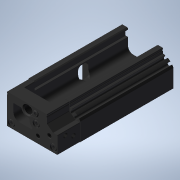
# Autodesk Inventor part: DGSL-12---(50-0-0-30-zr)
Saved by Autodesk Inventor 2021 (Build 250183000, 183)
## iProperties
Created: 2026-04-25
Part Number: DGSL-12---(50-0-0-30-zr)
Material: Generic
Catalog Web Link: www.3dfindit.com
Description: DGSL-(ZR)-Mini slide, cylinder
Vendor: FESTO
Document SubType Name: Modeling
Designer: psAdmin
Manufacturer: FESTO
Mass: 154.278 g
Surface Area: 450.594 cm^2
Volume: 154.278 cm^3
Density: 1 g/cm^3
Appearance: PSOLRGB-176-176-176
Category: PARTsolutions
Company: FESTO
Title: DGSL-12-50-0-0-3
Author: Cadenas PARTsolutions
Comments: Mini slide, cylinder
PSOL_IDENT_0: {$CADENAS_DATA/23d-libs/festo/parts/d/dgsl/parts/dgsl_zylinder.prj},221 {VTYP=3D},{NB=DGSL-12---(50-
PSOL_IDENT_1: 0-0-30-zr)},{LINA=DGSL-12-50-0-0-3},{NN=DGSL-(ZR)},{DATE=08.01.2026 09:23:11},{GEOMDATE=08.01.2026 0
PSOL_IDENT_2: 9:23:00},{VERSION=},{LINEID=110},{WBVAR=TYP2,HUB,FE,EL,DA,HGO},{WBNUMERIC=HUB,FE,EL,DA,HGO}  {NB=DGS
PSOL_IDENT_3: L-12---(50-0-0-30-zr)},{LINA=DGSL-12-50-0-0-3},{KT=DUMMY},{TYP=DGSL-12},{TYP2=},{TYP22=},{KDM=16},{E
PSOL_IDENT_4: E=M5},{KDM2=12},{PS=A},{ZB=24.000},{B4=34.000},{HUB=50},{FE=0},{EL=0},{DA=3},{OFFX=-0.500},{OFFY=-1.
PSOL_IDENT_5: 500},{LAOFF=0.500},{T1=8.700},{T11=14.000},{T1H=10.800},{T1R=4.000},{LA=10.000},{LA2=4.500},{LAN=5.0
PSOL_IDENT_6: 00},{LAH=1.600},{LAH2=5.600},{LAH3=11.300},{LAD1=7.000},{LAD2=9.000},{LAD3=5.500},{L=108.6},{LD=26.0
PSOL_IDENT_7: 00},{LD1=11.900},{B=59.000},{B0=45.100},{B1=23.800},{B1A=24.970},{B1B=9.250},{B2=36.700},{B3=50.000}
PSOL_IDENT_8: ,{B6=5.000},{H0=14.300},{H1=27.700},{H1A=27.800},{H1B=5.000},{H2=8.000},{H3=15.100},{H4=18.800},{H5=
PSOL_IDENT_9: 24.900},{H6=5.000},{H16=5.000},{L2=26.85},{L2P=26.900},{L2P1=25.700},{L2Y3=26.850},{L5=82.4},{L6=0},
PSOL_IDENT_10: {L7=0},{L8=12.000},{D1N=10},{D1B=9.100},{D2N=5.000},{D3N=5.000},{D4N=4.300},{D4N2=8.000},{D4HEX=3.00
PSOL_IDENT_11: 0},{D4HEXR=1.800},{D6A=8.000},{D6B=4.300},{KSD1=16.500},{KSD=6.000},{SH1=10.250},{SH2=15.250},{SL1=1
PSOL_IDENT_12: 8.5},{ST1=24.000},{ST11=5.500},{SDN1=5.000},{SL2=9.000},{ST2=12.800},{ST22=5.500},{SDN2=5.000},{E3H=
PSOL_IDENT_13: 14.800},{E3B=0},{E3B1=10.500},{E3B2=19.900},{E3L=10.300},{E3D=16.000},{E3X=0.500},{SDDNP=10.000},{SD
PSOL_IDENT_14: DNY3=10.000},{D1K=8.917},{D1P=1.000},{KPX=3.600},{KPL=18.000},{KPR=3.000},{KPH=24.000},{ANSOFF=0.500
PSOL_IDENT_15: },{SH=59.000},{KEH=10.600},{KEB=5.000},{KED=6.000},{KEN=6.000},{KENS=3.000},{KENT=2.000},{BND=3.000}
PSOL_IDENT_16: ,{BNT=6.000},{BNT2=8.000},{BNP=30.800},{BNP2=10.000},{FI=4.600},{FD=8.000},{FP1=54.000},{FP2=5.000},
PSOL_IDENT_17: {FP3=5.000},{DK=7.000},{K=4.000},{S=3.000},{T=2.000},{RD=4.600},{L100=1.200},{L101=9.500},{H101=14.6
PSOL_IDENT_18: 00},{L102=22.800},{H102=7.500},{L103=5.500},{L104=9.500},{L105=5.500},{L106=18.400},{L107=7.000},{L1
PSOL_IDENT_19: 08=9.400},{D107=4.000},{L109=6.000},{HUBSTOFF=1.600},{HUBCORR=1.600},{L110=5.000},{L111=3.000},{D111=
PSOL_IDENT_20: 8.080},{GEHL=60.000},{HGO=0},{SENX=49.203},{SENY=23.978},{SENX2=53.110},{SENY2=21.097},{SENW=153.500
PSOL_IDENT_21: },{SENW2=133.000}
NB: DGSL-12---(50-0-0-30-zr)
NN: DGSL-(ZR)
NT: Mini slide, cylinder
NBSYN: $TYP.$TYP22.---($HUB.-$FE.-$EL.-$DA.$HGO.-zr)
LINA: DGSL-12-50-0-0-3
CATALOG: Festo
TYP: DGSL-12
KDM: 16
EE: M5
ZB: 24
HUB: 50
FE: -
EL: -
DA: Y3
T11: 14
ST11: 5.5
ST22: 5.5
D1K: 8.917
D1P: 1
ANSOFF: 0.5
SH: 59
KEH: 10.6
KEB: 5
KED: 6
KEN: 6
KENS: 3
KENT: 2
BND: 3
BNT: 6
BNT2: 8
BNP: 30.8
BNP2: 10
FI: 4.6
FD: 8
FP1: 54
FP2: 5
FP3: 5
DK: 7
K: 4
S: 3
T: 2
RD: 4.6
L100: 1.2
L101: 9.5
H101: 14.6
L102: 22.8
H102: 7.5
L103: 5.5
L104: 9.5
L105: 5.5
L106: 18.4
L107: 7
L108: 9.4
D107: 4
L109: 6
HUBSTOFF: 1.6
L110: 5
L111: 3
D111: 8.08
GEHL: 60
HGO: 0
SENX: 49.203
SENY: 23.978
SENX2: 53.11
SENY2: 21.097
SENW: 153.5
SENW2: 133
SUPPLIER: FESTO
ARTICLENO: DGSL-12---(50-0-0-30-zr)
BOMINFO: DGSL-12-50-0-0-3
CREATOR: CADENAS GmbH
Autodesk Inventor part; units mm, degrees
sketch "Skizze_Deckelprofil_12" plane through (0, 0, 0) normal (0, 0, 1) x (1, 0, 0)
  arc A0 (0, 0.5) -> (0.5, 0) centre (0.5, 0.5) ccw
  line L0 (0.5, 0) -> (58.5, 0)
  arc A1 (58.5, 0) -> (59, 0.5) centre (58.5, 0.5) ccw
  line L1 (59, 0.5) -> (59, 19.35)
  arc A2 (59, 19.35) -> (58.5, 19.85) centre (58.5, 19.35) ccw
  line L2 (58.5, 19.85) -> (54.1325, 19.85)
  arc A3 (53.7137, 19.9891) -> (54.1325, 19.85) centre (54.1325, 20.55) ccw
  line L3 (53.7137, 19.9891) -> (46.8812, 25.0912)
  arc A4 (46.6, 25.6521) -> (46.8812, 25.0912) centre (47.3, 25.6521) ccw
  line L4 (46.6, 25.6521) -> (46.6, 31.5253)
  arc A5 (46.6, 31.5253) -> (46.5167, 31.6878) centre (46.4, 31.5253) ccw
  arc A6 (46.5167, 33.3122) -> (46.5167, 31.6878) centre (47.1, 32.5) ccw
  arc A7 (46.5167, 33.3122) -> (46.6, 33.4747) centre (46.4, 33.4747) ccw
  line L5 (46.6, 33.4747) -> (46.6, 34.2)
  arc A8 (46.6, 34.2) -> (46.1, 34.7) centre (46.1, 34.2) ccw
  line L6 (46.1, 34.7) -> (0.5, 34.7)
  arc A9 (0.5, 34.7) -> (0, 34.2) centre (0.5, 34.2) ccw
  line L7 (0, 34.2) -> (0, 33.4747)
  arc A10 (0, 33.4747) -> (0.0833, 33.3122) centre (0.2, 33.4747) ccw
  arc A11 (0.0833, 31.6878) -> (0.0833, 33.3122) centre (-0.5, 32.5) ccw
  arc A12 (0.0833, 31.6878) -> (0, 31.5253) centre (0.2, 31.5253) ccw
  line L8 (0, 31.5253) -> (0, 0.5)
  arc A13 (7.5, 17.8) -> (14.5, 10.8) centre (14.5, 17.8) ccw
  line L9 (14.5, 10.8) -> (28.9, 10.8)
  arc A14 (28.9, 10.8) -> (29.5, 11.4) centre (28.9, 11.4) ccw
  line L10 (29.5, 11.4) -> (29.5, 12.7814)
  arc A15 (29.5, 12.7814) -> (29.2417, 13.2746) centre (28.9, 12.7814) ccw
  arc A16 (26.4, 18.7) -> (29.2417, 13.2746) centre (33, 18.7) ccw
  line L11 (26.4, 18.7) -> (26.4, 19.8616)
  arc A17 (26.4, 19.8616) -> (25.2, 20.8414) centre (25.4, 19.8616) ccw
  arc A18 (16.9377, 26.3184) -> (25.2, 20.8414) centre (23.8, 27.7) ccw
  arc A19 (16.9377, 26.3184) -> (16.3495, 26.8) centre (16.3495, 26.2) ccw
  line L12 (16.3495, 26.8) -> (8.1, 26.8)
  arc A20 (8.1, 26.8) -> (7.5, 26.2) centre (8.1, 26.2) ccw
  line L13 (7.5, 26.2) -> (7.5, 17.8)
  constraints: 42 point on circle, 28 end point, 21 centre point
extrude "Extrusion1" add sketch "Skizze_Deckelprofil_12" along normal blind 26
sketch "Skizze_Gehaeuseprofil_12" plane through (0, 0, 0) normal (0, 0, 1) x (1, 0, 0)
  line L0 (-0.5, 0.3) -> (0, -0.2)
  line L1 (0, -0.2) -> (5.65, -0.2)
  line L2 (5.65, -0.2) -> (5.95, -0.5)
  line L3 (5.95, -0.5) -> (41.2, -0.5)
  line L4 (41.2, -0.5) -> (41.5, -0.2)
  line L5 (41.5, -0.2) -> (59, -0.2)
  line L6 (59, -0.2) -> (59.5, 0.3)
  line L7 (59.5, 0.3) -> (59.5, 20.9212)
  arc A0 (59.5, 20.9212) -> (59.4448, 21.1495) centre (59, 20.9212) ccw
  arc A1 (59.4448, 21.1495) -> (58.0866, 23.3179) centre (46.1, 14.3) ccw
  arc A2 (58.0866, 23.3179) -> (57.7956, 23.3486) centre (57.9268, 23.1976) ccw
  line L8 (57.7956, 23.3486) -> (56.2727, 22.0247)
  arc A3 (56.2727, 22.0247) -> (56.2529, 21.7426) centre (56.4039, 21.8738) ccw
  arc A4 (56.2155, 21.4467) -> (56.2529, 21.7426) centre (56.102, 21.6114) ccw
  line L9 (56.2155, 21.4467) -> (55.4047, 20.8876)
  arc A5 (53.0577, 23.5876) -> (55.4047, 20.8876) centre (54.3829, 22.3695) ccw
  line L10 (53.0577, 23.5876) -> (53.7241, 24.3127)
  arc A6 (54.0223, 24.3086) -> (53.7241, 24.3127) centre (53.8714, 24.1774) ccw
  arc A7 (54.0223, 24.3086) -> (54.3045, 24.2889) centre (54.1733, 24.4398) ccw
  line L11 (54.3045, 24.2889) -> (55.7128, 25.513)
  arc A8 (55.7128, 25.513) -> (55.7097, 25.8176) centre (55.5815, 25.664) ccw
  arc A9 (55.7097, 25.8176) -> (52.9206, 27.6596) centre (46.1, 14.3) ccw
  arc A10 (52.9206, 27.6596) -> (52.647, 27.5628) centre (52.8297, 27.4815) ccw
  line L12 (52.647, 27.5628) -> (51.9613, 26.0228)
  arc A11 (51.9613, 26.0228) -> (52.0626, 25.7587) centre (52.144, 25.9414) ccw
  arc A12 (52.1538, 25.4747) -> (52.0626, 25.7587) centre (51.9813, 25.576) ccw
  line L13 (52.1538, 25.4747) -> (51.6552, 24.6254)
  arc A13 (48.387, 26.0805) -> (51.6552, 24.6254) centre (50.1029, 25.5366) ccw
  line L14 (48.387, 26.0805) -> (48.6846, 27.0193)
  arc A14 (48.9566, 27.1416) -> (48.6846, 27.0193) centre (48.8752, 26.9589) ccw
  arc A15 (48.9566, 27.1416) -> (49.2206, 27.243) centre (49.0379, 27.3243) ccw
  line L15 (49.2206, 27.243) -> (49.8202, 28.5897)
  arc A16 (49.8202, 28.5897) -> (49.6853, 28.8652) centre (49.6375, 28.671) ccw
  arc A17 (49.6853, 28.8652) -> (47.3745, 29.2458) centre (46.1, 14.3) ccw
  arc A18 (47.1, 29.5447) -> (47.3745, 29.2458) centre (47.4, 29.5447) ccw
  line L16 (47.1, 29.5447) -> (47.1, 31.6225)
  arc A19 (47.1, 31.6225) -> (46.9444, 31.8175) centre (46.9, 31.6225) ccw
  arc A20 (46.9444, 33.1825) -> (46.9444, 31.8175) centre (47.1, 32.5) ccw
  arc A21 (46.9444, 33.1825) -> (47.1, 33.3775) centre (46.9, 33.3775) ccw
  line L17 (47.1, 33.3775) -> (47.1, 34.5)
  arc A22 (47.1, 34.5) -> (46.6, 35) centre (46.6, 34.5) ccw
  line L18 (46.6, 35) -> (41.7124, 35)
  line L19 (41.7124, 35) -> (40.5, 34.3)
  line L20 (40.5, 34.3) -> (40.5, 33)
  line L21 (40.5, 33) -> (43.45, 33)
  line L22 (43.45, 33) -> (43.45, 25.8)
  arc A23 (43.25, 25.6) -> (43.45, 25.8) centre (43.25, 25.8) ccw
  line L23 (43.25, 25.6) -> (40.695, 25.6)
  arc A24 (40.695, 25.6) -> (40.496, 25.38) centre (40.695, 25.4) ccw
  arc A25 (39.7, 24.5) -> (40.496, 25.38) centre (39.7, 25.3) ccw
  line L24 (39.7, 24.5) -> (33.5, 24.5)
  arc A26 (33.5, 24.5) -> (30, 21) centre (33.5, 21) ccw
  line L25 (30, 21) -> (30, 11.8)
  arc A27 (29, 10.8) -> (30, 11.8) centre (29, 11.8) ccw
  line L26 (29, 10.8) -> (12.5, 10.8)
  arc A28 (6.5, 16.8) -> (12.5, 10.8) centre (12.5, 16.8) ccw
  line L27 (6.5, 16.8) -> (6.5, 25.4)
  arc A29 (6.5, 25.4) -> (6.3, 25.6) centre (6.3, 25.4) ccw
  line L28 (6.3, 25.6) -> (3.75, 25.6)
  arc A30 (3.55, 25.8) -> (3.75, 25.6) centre (3.75, 25.8) ccw
  line L29 (3.55, 25.8) -> (3.55, 33)
  line L30 (3.55, 33) -> (6.5, 33)
  line L31 (6.5, 33) -> (6.5, 34.3)
  line L32 (6.5, 34.3) -> (5.2876, 35)
  line L33 (5.2876, 35) -> (0, 35)
  arc A31 (0, 35) -> (-0.5, 34.5) centre (0, 34.5) ccw
  line L34 (-0.5, 34.5) -> (-0.5, 33.3775)
  arc A32 (-0.5, 33.3775) -> (-0.3444, 33.1825) centre (-0.3, 33.3775) ccw
  arc A33 (-0.3444, 31.8175) -> (-0.3444, 33.1825) centre (-0.5, 32.5) ccw
  arc A34 (-0.3444, 31.8175) -> (-0.5, 31.6225) centre (-0.3, 31.6225) ccw
  line L35 (-0.5, 31.6225) -> (-0.5, 0.3)
  constraints: 72 end point, 70 point on circle, 35 centre point
extrude "Extrusion2" add sketch "Skizze_Gehaeuseprofil_12" against normal blind 108.6
sketch "Skizze_Deckelschnitt_12" plane through (0, 0, 0) normal (0, 0, 1) x (1, 0, 0)
  line L0 (6, 34.7) -> (6.5, 34.2)
  line L1 (6.5, 34.2) -> (6.5, 16.8)
  arc A0 (6.5, 16.8) -> (12.5, 10.8) centre (12.5, 16.8) ccw
  line L2 (12.5, 10.8) -> (28.5, 10.8)
  arc A1 (28.5, 10.8) -> (30, 16.3981) centre (28.5, 13.8) ccw
  line L3 (30, 16.3981) -> (30, 21)
  arc A2 (33.5, 24.5) -> (30, 21) centre (33.5, 21) ccw
  line L4 (33.5, 24.5) -> (39.5, 24.5)
  arc A3 (39.5, 24.5) -> (40.5, 30.3284) centre (39.5, 27.5) ccw
  line L5 (40.5, 30.3284) -> (40.5, 34.2)
  line L6 (40.5, 34.2) -> (41, 34.7)
  line L7 (41, 34.7) -> (6, 34.7)
  constraints: 16 end point, 8 point on circle, 4 centre point
extrude "Extrusion3" cut sketch "Skizze_Deckelschnitt_12" along normal blind 11.9
sketch "Skizze_Frontsenkung_1" plane through (0, 0, 26) normal (0, 0, 1) x (1, 0, 0)
  arc A0 (26.5913, 32.5116) -> (27.3844, 23.4462) centre (26.9878, 27.9789) ccw
  line L0 (27.3844, 23.4462) -> (33.4114, 23.9735)
  arc A1 (33.4114, 23.9735) -> (32.6182, 33.0389) centre (33.0148, 28.5062) ccw
  line L1 (32.6182, 33.0389) -> (26.5913, 32.5116)
  constraints: 4 end point, 4 point on circle, 2 centre point
extrude "Extrusion4" cut sketch "Skizze_Frontsenkung_1" against normal blind 6
sketch "Sketch_9" plane through (0, 0, 20) normal (0, 0, 1) x (1, 0, 0)
  line L0 (25.5951, 32.4244) -> (26.3882, 23.3591)
  line L1 (26.3882, 23.3591) -> (33.4114, 23.9735)
  arc A0 (33.4114, 23.9735) -> (32.6182, 33.0389) centre (33.0148, 28.5062) ccw
  line L2 (32.6182, 33.0389) -> (25.5951, 32.4244)
  constraints: 6 end point, 2 point on circle, 1 centre point
extrude "Extrusion5" add sketch "Sketch_9" along normal blind 5
sketch "Sketch_10" plane through (0, 27.7, 0) normal (0, 1, 0) x (1, 0, 0)
  line L0 (23.8, -25) -> (23.8, -20)
  line L1 (23.8, -20) -> (27.6, -20)
  line L2 (27.6, -20) -> (27.6, -23.8)
  line L3 (27.6, -23.8) -> (28.8, -25)
  line L4 (28.8, -25) -> (23.8, -25)
  line L5 (23.8, -25) -> (23.8, -20)
  constraints: 12 end point
revolve "Revolution1" cut sketch "Sketch_10" angle 360 about axis through (23.8, 27.7, 25) along (0, 0, 1)
sketch "Sketch_26" plane through (0, 0, 26) normal (0, 0, 1) x (1, 0, 0)
  arc A0 (23.3642, 32.681) -> (24.2358, 22.719) centre (23.8, 27.7) ccw
  line L0 (24.2358, 22.719) -> (27.4236, 22.9979)
  line L1 (27.4236, 22.9979) -> (27.3844, 23.4462)
  arc A1 (26.5913, 32.5116) -> (27.3844, 23.4462) centre (26.9878, 27.9789) ccw
  line L2 (26.5913, 32.5116) -> (26.552, 32.9599)
  line L3 (26.552, 32.9599) -> (23.3642, 32.681)
  constraints: 8 end point, 4 point on circle, 2 centre point
extrude "Extrusion6" add sketch "Sketch_26" against normal blind 6
sketch "Skizze_Frontbohrung_1" plane through (23.8, 0, 0) normal (1, 0, 0) x (0, 0, -1)
  line L0 (-26, 27.7) -> (-11.9, 27.7)
  line L1 (-11.9, 27.7) -> (-11.9, 23.2415)
  line L2 (-11.9, 23.2415) -> (-24.8, 23.2415)
  line L3 (-24.8, 23.2415) -> (-26, 22.0415)
  line L4 (-26, 22.0415) -> (-26, 27.7)
  line L5 (-26, 27.7) -> (-11.9, 27.7)
  constraints: 12 end point
revolve "Revolution2" cut sketch "Skizze_Frontbohrung_1" angle 360 about axis through (23.8, 27.7, 26) along (0, 0, 1)
thread "Thread1" size "M10x1" class "6H" standard "ISO Metric profile" length 12.9
sketch "Sketch9" plane through (0, 0, 26) normal (0, 0, 1) x (1, 0, 0)
  point P0 (36.2, 7.5)
hole "Hole1" at (36.2, 7.5, 26) direction (0, 0, -1) diameter 4.134 depth 18.4 tip angle 120 countersink diameter 5 countersink angle 90 thread size "M5x0.8" class "6H" standard "ISO Metric profile"
sketch "Sketch10" plane through (0, 0, 26) normal (0, 0, 1) x (1, 0, 0)
  point P0 (49.5, 14.6)
hole "Hole2" at (49.5, 14.6, 26) direction (0, 0, -1) diameter 4.134 depth 9.5 tip angle 120 countersink diameter 5 countersink angle 90 thread size "M5x0.8" class "6H" standard "ISO Metric profile"
sketch "Skizze_Anschlag_Cut_1" plane through (0, 0, 0) normal (1, 0, 0) x (0, 1, 0)
  line L0 (20.4, -50.4) -> (-0.5, -50.4)
  line L1 (-0.5, -50.4) -> (-0.5, -62.4)
  line L2 (-0.5, -62.4) -> (20.4, -62.4)
  arc A0 (20.4, -62.4) -> (24.4, -58.4) centre (20.4, -58.4) ccw
  line L3 (24.4, -58.4) -> (24.4, -54.4)
  arc A1 (24.4, -54.4) -> (20.4, -50.4) centre (20.4, -54.4) ccw
  constraints: 8 end point, 4 point on circle, 2 centre point
extrude "Extrusion7" cut sketch "Skizze_Anschlag_Cut_1" along normal mid plane 16.4
sketch "Skizze_Anschlag_Cut_1b" plane through (0, 0, 0) normal (1, 0, 0) x (0, 1, 0)
  arc A0 (14.8, -50.4) -> (10.8, -54.4) centre (14.8, -54.4) ccw
  line L0 (10.8, -54.4) -> (10.8, -58.4)
  arc A1 (10.8, -58.4) -> (14.8, -62.4) centre (14.8, -58.4) ccw
  line L1 (14.8, -62.4) -> (20.4, -62.4)
  arc A2 (20.4, -62.4) -> (24.4, -58.4) centre (20.4, -58.4) ccw
  line L2 (24.4, -58.4) -> (24.4, -54.4)
  arc A3 (24.4, -54.4) -> (20.4, -50.4) centre (20.4, -54.4) ccw
  line L3 (20.4, -50.4) -> (14.8, -50.4)
  constraints: 8 end point, 8 point on circle, 4 centre point
extrude "Extrusion8" cut sketch "Skizze_Anschlag_Cut_1b" along normal blind 14
sketch "Sketch13" plane through (59, 0.5, 26) normal (1, 0, 0) x (0, 0, -1)
  point P0 (18.5, 9.75)
hole "Hole3" at (59, 10.25, 7.5) direction (-1, 0, 0) diameter 4.134 depth 24 tip angle 120 countersink diameter 5 countersink angle 90 thread size "M5x0.8" class "6H" standard "ISO Metric profile"
sketch "Sketch14" plane through (59, 0.5, 26) normal (1, 0, 0) x (0, 0, -1)
  point P0 (9, 14.75)
hole "Hole4" at (59, 15.25, 17) direction (-1, 0, 0) diameter 4.134 depth 12.8 tip angle 120 countersink diameter 5 countersink angle 90 thread size "M5x0.8" class "6H" standard "ISO Metric profile"
sketch "Skizze_Zylinder_HUB_Deckel" plane through (45.1, 0, 0) normal (1, 0, 0) x (0, 0, -1)
  line L0 (108.6, 14.3) -> (40.2, 14.3)
  line L1 (40.2, 14.3) -> (40.2, 22.3)
  line L2 (40.2, 22.3) -> (100.2, 22.3)
  line L3 (100.2, 22.3) -> (100.2, 17.3)
  line L4 (100.2, 17.3) -> (105.6, 17.3)
  line L5 (105.6, 17.3) -> (105.6, 18.34)
  line L6 (105.6, 18.34) -> (108.6, 18.34)
  line L7 (108.6, 18.34) -> (108.6, 14.3)
  line L8 (108.6, 14.3) -> (40.2, 14.3)
  constraints: 18 end point
revolve "Revolution3" cut sketch "Skizze_Zylinder_HUB_Deckel" angle 360 about axis through (45.1, 14.3, -108.6) along (0, 0, -1)
sketch "Skizze_32" plane through (23.5, 0, 0) normal (1, 0, 0) x (0, 0, -1)
  line L0 (104.1, -0.5) -> (104.1, 10.8)
  line L1 (104.1, 10.8) -> (106.6, 10.8)
  line L2 (106.6, 10.8) -> (106.167, 10.367)
  line L3 (106.167, 10.367) -> (106.167, 1.533)
  line L4 (106.167, 1.533) -> (106.6, 1.1)
  line L5 (106.6, 1.1) -> (107.6, 1.1)
  line L6 (107.6, 1.1) -> (107.6, -0.5)
  line L7 (107.6, -0.5) -> (104.1, -0.5)
  line L8 (104.1, -0.5) -> (104.1, 10.8)
  constraints: 18 end point
revolve "Revolution4" cut sketch "Skizze_32" angle 360 about axis through (23.5, -0.5, -104.1) along (0, -1, 0)
thread "Thread2" size "M5x0.8" class "6H" standard "ISO Metric profile" full length
sketch "Skizze_33" plane through (23.5, 0, 0) normal (1, 0, 0) x (0, 0, -1)
  line L0 (94.1, -0.5) -> (94.1, 10.8)
  line L1 (94.1, 10.8) -> (96.6, 10.8)
  line L2 (96.6, 10.8) -> (96.167, 10.367)
  line L3 (96.167, 10.367) -> (96.167, 1.533)
  line L4 (96.167, 1.533) -> (96.6, 1.1)
  line L5 (96.6, 1.1) -> (97.6, 1.1)
  line L6 (97.6, 1.1) -> (97.6, -0.5)
  line L7 (97.6, -0.5) -> (94.1, -0.5)
  line L8 (94.1, -0.5) -> (94.1, 10.8)
  constraints: 18 end point
revolve "Revolution5" cut sketch "Skizze_33" angle 360 about axis through (23.5, -0.5, -94.1) along (0, -1, 0)
thread "Thread3" size "M5x0.8" class "6H" standard "ISO Metric profile" full length
sketch "Skizze_34" plane through (23.5, 0, 0) normal (1, 0, 0) x (0, 0, -1)
  line L0 (84.1, -0.5) -> (84.1, 15.8)
  line L1 (84.1, 15.8) -> (88.6, 15.8)
  line L2 (88.6, 15.8) -> (88.6, 5.1)
  line L3 (88.6, 5.1) -> (86.85, 5.1)
  line L4 (86.85, 5.1) -> (86.85, 1.1)
  line L5 (86.85, 1.1) -> (87.6, 1.1)
  line L6 (87.6, 1.1) -> (87.6, -0.5)
  line L7 (87.6, -0.5) -> (84.1, -0.5)
  line L8 (84.1, -0.5) -> (84.1, 15.8)
  constraints: 18 end point
revolve "Revolution6" cut sketch "Skizze_34" angle 360 about axis through (23.5, -0.5, -84.1) along (0, -1, 0)
sketch "Skizze_35" plane through (23.5, 0, 0) normal (1, 0, 0) x (0, 0, -1)
  line L0 (74.1, -0.5) -> (74.1, 15.8)
  line L1 (74.1, 15.8) -> (78.6, 15.8)
  line L2 (78.6, 15.8) -> (78.6, 5.1)
  line L3 (78.6, 5.1) -> (76.85, 5.1)
  line L4 (76.85, 5.1) -> (76.85, 1.1)
  line L5 (76.85, 1.1) -> (77.6, 1.1)
  line L6 (77.6, 1.1) -> (77.6, -0.5)
  line L7 (77.6, -0.5) -> (74.1, -0.5)
  line L8 (74.1, -0.5) -> (74.1, 15.8)
  constraints: 18 end point
revolve "Revolution7" cut sketch "Skizze_35" angle 360 about axis through (23.5, -0.5, -74.1) along (0, -1, 0)
sketch "Skizze_45" plane through (23.5, 0, 0) normal (1, 0, 0) x (0, 0, -1)
  line L0 (64.1, -0.5) -> (64.1, 15.8)
  line L1 (64.1, 15.8) -> (68.6, 15.8)
  line L2 (68.6, 15.8) -> (68.6, 5.1)
  line L3 (68.6, 5.1) -> (66.85, 5.1)
  line L4 (66.85, 5.1) -> (66.85, 1.1)
  line L5 (66.85, 1.1) -> (67.6, 1.1)
  line L6 (67.6, 1.1) -> (67.6, -0.5)
  line L7 (67.6, -0.5) -> (64.1, -0.5)
  line L8 (64.1, -0.5) -> (64.1, 15.8)
  constraints: 18 end point
revolve "Revolution8" cut sketch "Skizze_45" angle 360 about axis through (23.5, -0.5, -64.1) along (0, -1, 0)
sketch "Skizze_37" plane through (23.5, 0, 0) normal (1, 0, 0) x (0, 0, -1)
  line L0 (54.1, -0.5) -> (54.1, 10.8)
  line L1 (54.1, 10.8) -> (56.6, 10.8)
  line L2 (56.6, 10.8) -> (56.167, 10.367)
  line L3 (56.167, 10.367) -> (56.167, 1.533)
  line L4 (56.167, 1.533) -> (56.6, 1.1)
  line L5 (56.6, 1.1) -> (57.6, 1.1)
  line L6 (57.6, 1.1) -> (57.6, -0.5)
  line L7 (57.6, -0.5) -> (54.1, -0.5)
  line L8 (54.1, -0.5) -> (54.1, 10.8)
  constraints: 18 end point
revolve "Revolution9" cut sketch "Skizze_37" angle 360 about axis through (23.5, -0.5, -54.1) along (0, -1, 0)
thread "Thread4" size "M5x0.8" class "6H" standard "ISO Metric profile" full length
sketch "Skizze_36" plane through (23.5, 0, 0) normal (1, 0, 0) x (0, 0, -1)
  line L0 (44.1, -0.5) -> (44.1, 10.8)
  line L1 (44.1, 10.8) -> (46.6, 10.8)
  line L2 (46.6, 10.8) -> (46.167, 10.367)
  line L3 (46.167, 10.367) -> (46.167, 1.533)
  line L4 (46.167, 1.533) -> (46.6, 1.1)
  line L5 (46.6, 1.1) -> (47.6, 1.1)
  line L6 (47.6, 1.1) -> (47.6, -0.5)
  line L7 (47.6, -0.5) -> (44.1, -0.5)
  line L8 (44.1, -0.5) -> (44.1, 10.8)
  constraints: 18 end point
revolve "Revolution10" cut sketch "Skizze_36" angle 360 about axis through (23.5, -0.5, -44.1) along (0, -1, 0)
thread "Thread5" size "M5x0.8" class "6H" standard "ISO Metric profile" full length
sketch "Skizze_38" plane through (23.5, 0, 0) normal (1, 0, 0) x (0, 0, -1)
  line L0 (34.1, -0.5) -> (34.1, 15.8)
  line L1 (34.1, 15.8) -> (38.6, 15.8)
  line L2 (38.6, 15.8) -> (38.6, 5.1)
  line L3 (38.6, 5.1) -> (36.85, 5.1)
  line L4 (36.85, 5.1) -> (36.85, 1.1)
  line L5 (36.85, 1.1) -> (37.6, 1.1)
  line L6 (37.6, 1.1) -> (37.6, -0.5)
  line L7 (37.6, -0.5) -> (34.1, -0.5)
  line L8 (34.1, -0.5) -> (34.1, 15.8)
  constraints: 18 end point
revolve "Revolution11" cut sketch "Skizze_38" angle 360 about axis through (23.5, -0.5, -34.1) along (0, -1, 0)
sketch "Skizze_39" plane through (23.5, 0, 0) normal (1, 0, 0) x (0, 0, -1)
  line L0 (24.1, -0.5) -> (24.1, 15.8)
  line L1 (24.1, 15.8) -> (28.6, 15.8)
  line L2 (28.6, 15.8) -> (28.6, 5.1)
  line L3 (28.6, 5.1) -> (26.85, 5.1)
  line L4 (26.85, 5.1) -> (26.85, 1.1)
  line L5 (26.85, 1.1) -> (27.6, 1.1)
  line L6 (27.6, 1.1) -> (27.6, -0.5)
  line L7 (27.6, -0.5) -> (24.1, -0.5)
  line L8 (24.1, -0.5) -> (24.1, 15.8)
  constraints: 18 end point
revolve "Revolution12" cut sketch "Skizze_39" angle 360 about axis through (23.5, -0.5, -24.1) along (0, -1, 0)
sketch "Skizze_46" plane through (23.5, 0, 0) normal (1, 0, 0) x (0, 0, -1)
  line L0 (14.1, -0.5) -> (14.1, 15.8)
  line L1 (14.1, 15.8) -> (18.6, 15.8)
  line L2 (18.6, 15.8) -> (18.6, 5.1)
  line L3 (18.6, 5.1) -> (16.85, 5.1)
  line L4 (16.85, 5.1) -> (16.85, 1.1)
  line L5 (16.85, 1.1) -> (17.6, 1.1)
  line L6 (17.6, 1.1) -> (17.6, -0.5)
  line L7 (17.6, -0.5) -> (14.1, -0.5)
  line L8 (14.1, -0.5) -> (14.1, 15.8)
  constraints: 18 end point
revolve "Revolution13" cut sketch "Skizze_46" angle 360 about axis through (23.5, -0.5, -14.1) along (0, -1, 0)
sketch "Sketch_12" plane through (0, 0, 26) normal (0, 0, 1) x (1, 0, 0)
  circle A0 centre (54, 5) radius 4
  constraints: 1 centre point
extrude "Extrusion9" cut sketch "Sketch_12" along normal mid plane 9.2
sketch "Sketch_13" plane through (0, 0, 26) normal (0, 0, 1) x (1, 0, 0)
  circle A0 centre (5, 5) radius 4
  constraints: 1 centre point
extrude "Extrusion10" cut sketch "Sketch_13" along normal mid plane 9.2
sketch "Sketch_16" plane through (0, 0, 26) normal (0, 0, 1) x (1, 0, 0)
  circle A0 centre (34, 18.8) radius 4
  constraints: 1 centre point
extrude "Extrusion11" cut sketch "Sketch_16" along normal mid plane 9.2
sketch "Sketch_14" plane through (5, 0, 0) normal (1, 0, 0) x (0, 0, -1)
  line L0 (-21.4, 5) -> (-25.4, 5)
  line L1 (-25.4, 5) -> (-25.4, 7.9286)
  line L2 (-25.4, 7.9286) -> (-24.8286, 8.5)
  line L3 (-24.8286, 8.5) -> (-21.4, 8.5)
  line L4 (-21.4, 8.5) -> (-21.4, 5)
  line L5 (-21.4, 5) -> (-25.4, 5)
  constraints: 12 end point
revolve "Revolution14" add sketch "Sketch_14" angle 360 about axis through (5, 5, 21.4) along (0, 0, -1)
sketch "Sketch_7" plane through (33.0148, 0, 0) normal (1, 0, 0) x (0, 0, -1)
  line L0 (-26, 28.5062) -> (-20, 28.5062)
  line L1 (-20, 28.5062) -> (-20, 25.5062)
  line L2 (-20, 25.5062) -> (-25.4, 25.5062)
  line L3 (-25.4, 25.5062) -> (-26, 26.1062)
  line L4 (-26, 26.1062) -> (-26, 28.5062)
  line L5 (-26, 28.5062) -> (-20, 28.5062)
  constraints: 12 end point
sketch "Sketch_28" plane through (33.0148, 0, 0) normal (1, 0, 0) x (0, 0, -1)
  line L0 (-27, 28.5062) -> (-21, 28.5062)
  line L1 (-21, 28.5062) -> (-21, 25.5062)
  line L2 (-21, 25.5062) -> (-27, 25.5062)
  line L3 (-27, 25.5062) -> (-27, 28.5062)
  line L4 (-27, 28.5062) -> (-21, 28.5062)
  constraints: 10 end point
revolve "Revolution15" cut sketch "Sketch_28" angle 360 about axis through (33.0148, 28.5062, 27) along (0, 0, 1)
revolve "Revolution16" add sketch "Sketch_7" angle 360 about axis through (33.0148, 28.5062, 26) along (0, 0, 1)
sketch "Sketch_29" plane through (0, 0, 26) normal (0, 0, 1) x (1, 0, 0)
  line L0 (31.5148, 27.6402) -> (33.0148, 26.7741)
  line L1 (33.0148, 26.7741) -> (34.5148, 27.6402)
  line L2 (34.5148, 27.6402) -> (34.5148, 29.3722)
  line L3 (34.5148, 29.3722) -> (33.0148, 30.2382)
  line L4 (33.0148, 30.2382) -> (31.5148, 29.3722)
  line L5 (31.5148, 29.3722) -> (31.5148, 27.6402)
  constraints: 12 end point
extrude "Extrusion12" cut sketch "Sketch_29" against normal blind 2
sketch "Sketch33" plane through (0, 0.5, 26) normal (-1, 0, 0) x (0, 0, 1)
  point P0 (-10, 30.3)
hole "Hole5" at (0, 30.8, 16) direction (1, 0, 0) diameter 2.459 depth 8 tip angle 120 countersink diameter 3 countersink angle 90 thread size "M3x0.5" class "6H" standard "ISO Metric profile"
sketch "Sketch_15" plane through (34, 0, 0) normal (1, 0, 0) x (0, 0, -1)
  line L0 (-21.4, 18.8) -> (-25.4, 18.8)
  line L1 (-25.4, 18.8) -> (-25.4, 21.7286)
  line L2 (-25.4, 21.7286) -> (-24.8286, 22.3)
  line L3 (-24.8286, 22.3) -> (-21.4, 22.3)
  line L4 (-21.4, 22.3) -> (-21.4, 18.8)
  line L5 (-21.4, 18.8) -> (-25.4, 18.8)
  constraints: 12 end point
revolve "Revolution17" add sketch "Sketch_15" angle 360 about axis through (34, 18.8, 21.4) along (0, 0, -1)
sketch "Sketch_19" plane through (54, 0, 0) normal (1, 0, 0) x (0, 0, -1)
  line L0 (-21.4, 5) -> (-25.4, 5)
  line L1 (-25.4, 5) -> (-25.4, 7.9286)
  line L2 (-25.4, 7.9286) -> (-24.8286, 8.5)
  line L3 (-24.8286, 8.5) -> (-21.4, 8.5)
  line L4 (-21.4, 8.5) -> (-21.4, 5)
  line L5 (-21.4, 5) -> (-25.4, 5)
  constraints: 12 end point
revolve "Revolution18" add sketch "Sketch_19" angle 360 about axis through (54, 5, 21.4) along (0, 0, -1)
sketch "Sketch_20" plane through (0, 0, 25.4) normal (0, 0, 1) x (1, 0, 0)
  line L0 (52.5, 4.134) -> (54, 3.2679)
  line L1 (54, 3.2679) -> (55.5, 4.134)
  line L2 (55.5, 4.134) -> (55.5, 5.866)
  line L3 (55.5, 5.866) -> (54, 6.7321)
  line L4 (54, 6.7321) -> (52.5, 5.866)
  line L5 (52.5, 5.866) -> (52.5, 4.134)
  constraints: 12 end point
extrude "Extrusion13" cut sketch "Sketch_20" along normal mid plane 4
sketch "Sketch_21" plane through (0, 0, 25.4) normal (0, 0, 1) x (1, 0, 0)
  line L0 (3.5, 4.134) -> (5, 3.2679)
  line L1 (5, 3.2679) -> (6.5, 4.134)
  line L2 (6.5, 4.134) -> (6.5, 5.866)
  line L3 (6.5, 5.866) -> (5, 6.7321)
  line L4 (5, 6.7321) -> (3.5, 5.866)
  line L5 (3.5, 5.866) -> (3.5, 4.134)
  constraints: 12 end point
extrude "Extrusion14" cut sketch "Sketch_21" along normal mid plane 4
sketch "Sketch38" plane through (8.2, 0, 0) normal (-1, 0, 0) x (0, 0, 1)
  point P0 (-56.4, 5)
hole "Hole6" at (8.2, 5, -56.4) direction (1, 0, 0) diameter 3.242 depth 9.4 tip angle 120 countersink diameter 4 countersink angle 90 thread size "M4x0.7" class "6H" standard "ISO Metric profile"
sketch "Sketch_5" plane through (0, 0, 25.4) normal (0, 0, 1) x (1, 0, 0)
  line L0 (32.5, 17.934) -> (34, 17.0679)
  line L1 (34, 17.0679) -> (35.5, 17.934)
  line L2 (35.5, 17.934) -> (35.5, 19.666)
  line L3 (35.5, 19.666) -> (34, 20.5321)
  line L4 (34, 20.5321) -> (32.5, 19.666)
  line L5 (32.5, 19.666) -> (32.5, 17.934)
  constraints: 12 end point
extrude "Extrusion15" cut sketch "Sketch_5" along normal mid plane 4
ref_plane "ANBAU_XY" through (23.5, -0.5, -108.6) normal (0, 0, -1) x (-1, 0, 0)
ref_plane "ANBAU_YZ" through (23.5, -0.5, -108.6) normal (-1, 0, 0) x (0, 1, 0)
ref_plane "ANBAU_ZX" through (23.5, -0.5, -108.6) normal (0, 1, 0) x (0, 0, -1)
ref_plane "ANBAU_OLD_XY" through (22.55, 0, 0) normal (0, 0, -1) x (1, 0, 0)
ref_plane "ANBAU_OLD_YZ" through (22.55, 0, 0) normal (1, 0, 0) x (0, -1, 0)
ref_plane "ANBAU_OLD_ZX" through (22.55, 0, 0) normal (0, -1, 0) x (0, 0, -1)
ref_plane "CSL1_4_1_XY" through (23.5, 1.1, -104.1) normal (1, 0, 0) x (0, 0, -1)
ref_plane "CSL1_4_1_YZ" through (23.5, 1.1, -104.1) normal (0, 0, -1) x (0, 1, 0)
ref_plane "CSL1_4_1_ZX" through (23.5, 1.1, -104.1) normal (0, 1, 0) x (1, 0, 0)
ref_plane "CSL1_4_2_XY" through (23.5, 1.1, -94.1) normal (1, 0, 0) x (0, 0, -1)
ref_plane "CSL1_4_2_YZ" through (23.5, 1.1, -94.1) normal (0, 0, -1) x (0, 1, 0)
ref_plane "CSL1_4_2_ZX" through (23.5, 1.1, -94.1) normal (0, 1, 0) x (1, 0, 0)
ref_plane "FDT_DADS_XY" through (-0.5, 30.8, 16) normal (-1, 0, 0) x (0, 0, -1)
ref_plane "FDT_DADS_YZ" through (-0.5, 30.8, 16) normal (0, 0, -1) x (0, -1, 0)
ref_plane "FDT_DADS_ZX" through (-0.5, 30.8, 16) normal (0, -1, 0) x (-1, 0, 0)
ref_plane "FDT_QS_FRONT_IN_XY" through (36.2, 7.5, 26) normal (0, 0, 1) x (1, 0, 0)
ref_plane "FDT_QS_FRONT_IN_YZ" through (36.2, 7.5, 26) normal (1, 0, 0) x (0, 1, 0)
ref_plane "FDT_QS_FRONT_IN_ZX" through (36.2, 7.5, 26) normal (0, 1, 0) x (0, 0, 1)
ref_plane "FDT_QS_FRONT_OUT_XY" through (49.5, 14.6, 26) normal (0, 0, 1) x (1, 0, 0)
ref_plane "FDT_QS_FRONT_OUT_YZ" through (49.5, 14.6, 26) normal (1, 0, 0) x (0, 1, 0)
ref_plane "FDT_QS_FRONT_OUT_ZX" through (49.5, 14.6, 26) normal (0, 1, 0) x (0, 0, 1)
ref_plane "FDT_QS_SIDE_IN_XY" through (59, 10.25, 7.5) normal (1, 0, 0) x (0, 0, -1)
ref_plane "FDT_QS_SIDE_IN_YZ" through (59, 10.25, 7.5) normal (0, 0, -1) x (0, 1, 0)
ref_plane "FDT_QS_SIDE_IN_ZX" through (59, 10.25, 7.5) normal (0, 1, 0) x (1, 0, 0)
ref_plane "FDT_QS_SIDE_OUT_XY" through (59, 15.25, 17) normal (1, 0, 0) x (0, 0, -1)
ref_plane "FDT_QS_SIDE_OUT_YZ" through (59, 15.25, 17) normal (0, 0, -1) x (0, 1, 0)
ref_plane "FDT_QS_SIDE_OUT_ZX" through (59, 15.25, 17) normal (0, 1, 0) x (1, 0, 0)
ref_plane "FDT_SEN11_XY" through (49.203, 23.978, -54.3) normal (0.4461978, 0.8949344, 0) x (-0.8949344, 0.4461978, 0)
ref_plane "FDT_SEN11_YZ" through (49.203, 23.978, -54.3) normal (-0.8949344, 0.4461978, 0) x (0, 0, 1)
ref_plane "FDT_SEN11_ZX" through (49.203, 23.978, -54.3) normal (0, 0, 1) x (0.4461978, 0.8949344, 0)
ref_plane "FDT_SEN21_XY" through (53.11, 21.097, -54.3) normal (0.7313537, 0.6819984, 0) x (-0.6819984, 0.7313537, 0)
ref_plane "FDT_SEN21_YZ" through (53.11, 21.097, -54.3) normal (-0.6819984, 0.7313537, 0) x (0, 0, 1)
ref_plane "FDT_SEN21_ZX" through (53.11, 21.097, -54.3) normal (0, 0, 1) x (0.7313537, 0.6819984, 0)
ref_plane "IP_A1_XY" through (8.2, 5, -56.4) normal (1, 0, 0) x (0, 0, -1)
ref_plane "IP_A1_YZ" through (8.2, 5, -56.4) normal (0, 0, -1) x (0, 1, 0)
ref_plane "IP_A1_ZX" through (8.2, 5, -56.4) normal (0, 1, 0) x (1, 0, 0)
ref_plane "IP_A2_XY" through (8.2, 5, -56.4) normal (1, 0, 0) x (0, 0, -1)
ref_plane "IP_A2_YZ" through (8.2, 5, -56.4) normal (0, 0, -1) x (0, 1, 0)
ref_plane "IP_A2_ZX" through (8.2, 5, -56.4) normal (0, 1, 0) x (1, 0, 0)
ref_plane "IP_A3_XY" through (8.2, 5, -56.4) normal (1, 0, 0) x (0, 0, -1)
ref_plane "IP_A3_YZ" through (8.2, 5, -56.4) normal (0, 0, -1) x (0, 1, 0)
ref_plane "IP_A3_ZX" through (8.2, 5, -56.4) normal (0, 1, 0) x (1, 0, 0)
ref_plane "IP_BS_1_XY" through (36.2, 7.5, 26) normal (0, 0, -1) x (1, 0, 0)
ref_plane "IP_BS_1_YZ" through (36.2, 7.5, 26) normal (1, 0, 0) x (0, -1, 0)
ref_plane "IP_BS_1_ZX" through (36.2, 7.5, 26) normal (0, -1, 0) x (0, 0, -1)
ref_plane "IP_BS_2_XY" through (49.5, 14.6, 26) normal (0, 0, -1) x (1, 0, 0)
ref_plane "IP_BS_2_YZ" through (49.5, 14.6, 26) normal (1, 0, 0) x (0, -1, 0)
ref_plane "IP_BS_2_ZX" through (49.5, 14.6, 26) normal (0, -1, 0) x (0, 0, -1)
ref_plane "IP_KS_XY" through (45.1, 14.3, -40.2) normal (0, 0, -1) x (1, 0, 0)
ref_plane "IP_KS_YZ" through (45.1, 14.3, -40.2) normal (1, 0, 0) x (0, -1, 0)
ref_plane "IP_KS_ZX" through (45.1, 14.3, -40.2) normal (0, -1, 0) x (0, 0, -1)
ref_plane "IP_SA_1_XY" through (59, 15.25, 17) normal (-1, 0, 0) x (0, 0, -1)
ref_plane "IP_SA_1_YZ" through (59, 15.25, 17) normal (0, 0, -1) x (0, -1, 0)
ref_plane "IP_SA_1_ZX" through (59, 15.25, 17) normal (0, -1, 0) x (-1, 0, 0)
ref_plane "IP_SA_2_XY" through (59, 10.25, 7.5) normal (-1, 0, 0) x (0, 0, -1)
ref_plane "IP_SA_2_YZ" through (59, 10.25, 7.5) normal (0, 0, -1) x (0, -1, 0)
ref_plane "IP_SA_2_ZX" through (59, 10.25, 7.5) normal (0, -1, 0) x (-1, 0, 0)
ref_plane "IP_SD_XY" through (23.8, 27.7, 26) normal (0, 0, 1) x (1, 0, 0)
ref_plane "IP_SD_YZ" through (23.8, 27.7, 26) normal (1, 0, 0) x (0, 1, 0)
ref_plane "IP_SD_ZX" through (23.8, 27.7, 26) normal (0, 1, 0) x (0, 0, 1)
ref_plane "SEN11_XY" through (49.203, 23.978, -10) normal (0, 0, -1) x (-0.8949344, 0.4461978, 0)
ref_plane "SEN11_YZ" through (49.203, 23.978, -10) normal (-0.8949344, 0.4461978, 0) x (0.4461978, 0.8949344, 0)
ref_plane "SEN11_ZX" through (49.203, 23.978, -10) normal (0.4461978, 0.8949344, 0) x (0, 0, -1)
ref_plane "SEN21_XY" through (53.11, 21.097, -86.65) normal (0, 0, -1) x (-0.6819984, 0.7313537, 0)
ref_plane "SEN21_YZ" through (53.11, 21.097, -86.65) normal (-0.6819984, 0.7313537, 0) x (0.7313537, 0.6819984, 0)
ref_plane "SEN21_ZX" through (53.11, 21.097, -86.65) normal (0.7313537, 0.6819984, 0) x (0, 0, -1)
body "Solid1"
